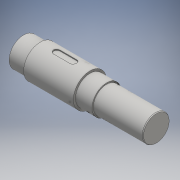
# Autodesk Inventor part: Shaft1
Saved by Autodesk Inventor 2016 (Build 200138000, 138)
## iProperties
Created: 2017-05-17
Part Number: Shaft1
Material: Типовые
Document SubType Name: Modeling
Designer: Admin
Density: 1 g/cm^3
Appearance: По умолчанию
Author: Admin
Autodesk Inventor part; units mm, degrees
ref_plane "YZ Plane" through (0, 0, 0) normal (1, 0, 0) x (0, 1, 0)
sketch "Эскиз1" plane through (0, 0, 0) normal (0, 0, 1) x (1, 0, 0)
  line L0 (0, 0) -> (-160, 0)
  line L1 (0, 0) -> (0, 15.4226)
  line L2 (0, 15.4226) -> (-1, 16)
  line L3 (-1, 16) -> (-60, 16)
  line L4 (-60, 16) -> (-60, 17.5)
  line L5 (-60, 17.5) -> (-80, 17.5)
  line L6 (-80, 17.5) -> (-80, 20)
  line L7 (-80, 20) -> (-140, 20)
  line L8 (-140, 20) -> (-140, 17.5)
  line L9 (-140, 17.5) -> (-160, 17.5)
  line L10 (-160, 17.5) -> (-160, 0)
  dimension "d0" = 160
  dimension "d1" = 32
  dimension "d2" = 30
  dimension "d3" = 1
  dimension "d4" = 60
  dimension "d5" = 35
  dimension "d6" = 20
  dimension "d7" = 40
  constraints: 22 end point, 7 perpendicular, 2 point on line, 1 collinear, 1 horizontal, 1 vertical
  measures "d0" distance of L0.start L0.end
  measures "d1" diameter of L3 L0
  measures "d2" angle of L3 L2
  measures "d3" horizontal distance of L2.end L1.end
  measures "d4" distance of L6.end L7.end
  measures "d5" diameter of L5 L0
  measures "d6" distance of L4.end L5.end
  measures "d7" diameter of L7 L0
revolve "Вращение1" add sketch "Эскиз1" angle 360 about axis through (0, 0, 0) along (-1, 0, 0)
ref_plane "РабПлоскость1" through (0, 14.5, 0) normal (0, 1, 0) x (-1, 0, 0)
ref_plane "РабПлоскость2" through (0, 0, 18.5) normal (0, 0, 1) x (1, 0, 0)
sketch "Эскиз3" plane through (0, 14.5, 0) normal (0, 1, 0) x (-1, 0, 0)
  line L0 (0, 15.4226) -> (0, -15.4226) projected
  line L1 (80, 20) -> (80, -20) projected
  line L2 (140, 20) -> (140, -20) projected
  line L3 (44, 0) -> (16, 0) construction
  line L4 (40, 4) -> (20, 4)
  line L5 (20, -4) -> (40, -4)
  arc A0 (40, -4) -> (40, 4) centre (40, 0) ccw
  arc A1 (20, 4) -> (20, -4) centre (20, 0) ccw
  point P0 (0, 0)
  point P1 (30, 0)
  point P2 (80, 0)
  dimension "d11" = 20
  dimension "d12" = 8
  dimension "d13" = 50
  constraints: 8 end point, 6 point on circle, 4 tangent, 2 centre point, 2 midpoint, 2 point on line, 1 horizontal, 1 horizontal alignment, 1 parallel
  measures "d11" distance of A1.centre A0.centre
  measures "d12" distance between parallel lines of L4 L5
  measures "d13" distance from line of L1 point (30, 0)
extrude "Выдавливание1" cut sketch "Эскиз3" along normal through all
sketch "Эскиз4" plane through (0, 0, 18.5) normal (0, 0, 1) x (1, 0, 0)
  line L0 (-124, 0) -> (-96, 0) construction
  line L1 (-120, -4) -> (-100, -4)
  line L2 (-100, 4) -> (-120, 4)
  arc A0 (-120, 4) -> (-120, -4) centre (-120, 0) ccw
  arc A1 (-100, -4) -> (-100, 4) centre (-100, 0) ccw
  line L3 (-80, -17.5) -> (-80, 17.5) projected
  point P0 (0, 0)
  point P1 (-110, 0)
  point P2 (-80, 0)
  dimension "d16" = 20
  dimension "d17" = 8
  dimension "d18" = 30
  constraints: 8 end point, 6 point on circle, 4 tangent, 2 centre point, 2 midpoint, 2 point on line, 1 horizontal, 1 horizontal alignment, 1 parallel
  measures "d16" distance of A1.centre A0.centre
  measures "d17" distance between parallel lines of L2 L1
  measures "d18" distance from line of L3 point (-110, 0)
extrude "Выдавливание2" cut sketch "Эскиз4" along normal through all
